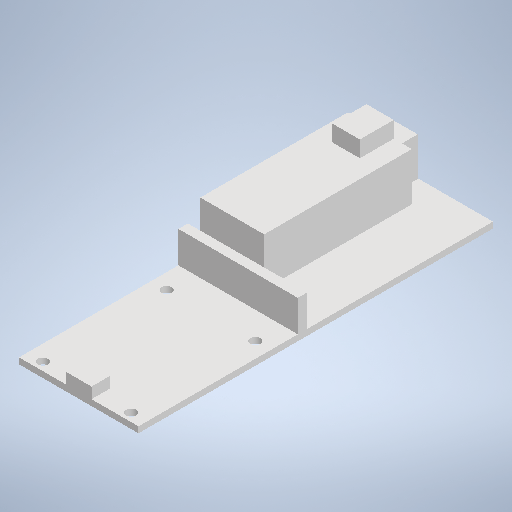
# Autodesk Inventor part: PCB Board
Saved by Autodesk Inventor 2025 (Build 290162000, 162)
## iProperties
Created: 2024-07-09
Part Number: PCB Board
Material: Generic
Document SubType Name: Modeling
Designer: track
Density: 1 g/cm^3
Appearance: Default
Author: track
Autodesk Inventor part; units mm, degrees
ref_plane "YZ Plane" through (0, 0, 0) normal (1, 0, 0) x (0, 1, 0)
ref_plane "XZ Plane" through (0, 0, 0) normal (0, 1, 0) x (-1, 0, 0)
ref_plane "XY Plane" through (0, 0, 0) normal (0, 0, 1) x (1, 0, 0)
sketch "Sketch1" plane through (0, 0, 0) normal (0, 1, 0) x (-1, 0, 0)
  line L0 (16.375, 48.6) -> (-16.375, 48.6)
  line L1 (-16.375, 48.6) -> (-16.375, -48.6)
  line L2 (-16.375, -48.6) -> (16.375, -48.6)
  line L3 (16.375, -48.6) -> (16.375, 48.6)
  line L4 (16.375, 48.6) -> (-16.375, -48.6) construction
  line L5 (-16.375, 48.6) -> (16.375, -48.6) construction
  point P0 (0, 0)
  dimension "d0" = 32.75
  dimension "d1" = 97.2
  constraints: 12 end point, 2 midpoint, 2 parallel, 1 horizontal, 1 perpendicular
  measures "d0" distance of L0.start L0.end
  measures "d1" distance of L0.end L1.end
extrude "Extrusion1" add sketch "Sketch1" along normal blind 1.65
sketch "Sketch3" plane through (0, 1.65, 0) normal (0, 1, 0) x (1, 0, 0)
  line L0 (-16.375, 48.6) -> (-16.375, -48.6) projected
  line L1 (-16.375, 41.6) -> (1.125, 41.6)
  line L2 (1.125, 41.6) -> (1.125, 1.1)
  line L3 (1.125, 1.1) -> (-16.375, 1.1)
  line L4 (-16.375, 1.1) -> (-16.375, 41.6)
  line L5 (16.375, 48.6) -> (-16.375, 48.6) projected
  point P0 (0, 0)
  dimension "d7" = 17.5
  dimension "d8" = 40.5
  dimension "d9" = 7
  constraints: 8 end point, 2 parallel, 1 horizontal, 1 perpendicular, 1 point on line
  measures "d7" distance of L1.start L1.end
  measures "d8" distance of L1.end L2.end
  measures "d9" distance between parallel lines of L5 L1
extrude "Extrusion3" add sketch "Sketch3" along normal blind 13.1
sketch "Sketch4" plane through (0, 1.65, 0) normal (0, 1, 0) x (1, 0, 0)
  line L0 (-16.375, 41.6) -> (1.125, 41.6) projected
  line L1 (-4.075, 41.6) -> (-11.075, 41.6)
  line L2 (-11.075, 41.6) -> (-11.075, 48.4118)
  line L3 (-11.075, 48.4118) -> (-4.075, 48.4118)
  line L4 (-4.075, 48.4118) -> (-4.075, 41.6)
  line L5 (-16.375, 48.6) -> (-16.375, 41.6) projected
  point P0 (0, 0)
  dimension "d12" = 7
  dimension "d13" = 5.3
  constraints: 8 end point, 2 parallel, 1 horizontal, 1 perpendicular, 1 point on line
  measures "d12" distance of L2.end L3.end
  measures "d13" distance between parallel lines of L5 L2
extrude "Extrusion4" add sketch "Sketch4" along normal blind 10.6
sketch "Sketch5" plane through (0, 14.75, 0) normal (0, 1, 0) x (1, 0, 0)
  line L0 (1.125, 41.6) -> (-16.375, 41.6) projected
  line L1 (-16.375, 41.6) -> (-16.375, 1.1) projected
  line L2 (-16.375, 1.1) -> (1.125, 1.1) projected
  line L3 (1.125, 1.1) -> (1.125, 41.6) projected
  line L4 (-11.075, 48.4118) -> (-11.075, 41.6) projected
  line L5 (-4.075, 41.6) -> (-11.075, 41.6) projected
  line L6 (-4.075, 41.6) -> (-4.075, 48.4118) projected
  line L7 (-4.075, 48.4118) -> (-11.075, 48.4118) projected
  line L8 (-4.075, 41.6) -> (-11.075, 41.6) projected
  line L9 (-3.825, 41.6) -> (-11.325, 41.6)
  line L10 (-11.325, 41.6) -> (-11.325, 32.3)
  line L11 (-11.325, 32.3) -> (-3.825, 32.3)
  line L12 (-3.825, 32.3) -> (-3.825, 41.6)
  point P0 (0, 0)
  point P1 (-7.575, 41.6)
  dimension "d16" = 9.3
  dimension "d17" = 7.5
  constraints: 8 end point, 2 midpoint, 2 parallel, 1 horizontal, 1 perpendicular, 1 point on line
  measures "d16" distance of L11.end L9.start
  measures "d17" distance of L10.end L11.end
extrude "Extrusion5" add sketch "Sketch5" along normal blind 4.46 contours L12 L11 L10 L0
sketch "Sketch6" plane through (-4.075, 1.65, -48.4118) normal (0, 0, -1) x (-1, 0, 0)
  point P0 (-4.075, -1.65)
sketch "Sketch7" plane through (0, 1.65, 0) normal (0, 1, 0) x (1, 0, 0)
  line L0 (-11.325, 32.3) -> (-11.325, 41.6) projected
  line L1 (-11.325, 41.6) -> (-16.375, 41.6) projected
  line L2 (-16.375, 41.6) -> (-16.375, 1.1) projected
  line L3 (-16.375, 1.1) -> (1.125, 1.1) projected
  line L4 (1.125, 1.1) -> (1.125, 41.6) projected
  line L5 (1.125, 41.6) -> (-3.825, 41.6) projected
  line L6 (-3.825, 41.6) -> (-3.825, 32.3) projected
  line L7 (-3.825, 32.3) -> (-11.325, 32.3) projected
  line L8 (16.375, -48.6) -> (16.375, 48.6) projected
  line L9 (-16.375, 48.6) -> (-16.375, -48.6) projected
  line L10 (16.375, -2.3) -> (-16.375, -2.3)
  line L11 (-16.375, -2.3) -> (-16.375, -4.9)
  line L12 (-16.375, -4.9) -> (16.375, -4.9)
  line L13 (16.375, -4.9) -> (16.375, -2.3)
  point P0 (0, 0)
  point P1 (-16.375, -2.3)
  dimension "d20" = 2.6
  dimension "d21" = 3.4
  constraints: 8 end point, 2 parallel, 2 point on line, 1 horizontal, 1 perpendicular
  measures "d20" distance between parallel lines of L10 L12
  measures "d21" distance between parallel lines of L3 L10
extrude "Extrusion6" add sketch "Sketch7" along normal blind 8.65 contours L10 L8 L12 L9
sketch "Sketch8" plane through (0, 1.65, 0) normal (0, 1, 0) x (1, 0, 0)
  circle A0 centre (-12.125, -46.35) radius 1.4
  line L0 (-16.375, -4.9) -> (-16.375, -48.6) projected
  line L1 (-16.375, -48.6) -> (16.375, -48.6) projected
  circle A1 centre (-12.125, -12.35) radius 1.4
  line L2 (0, -48.6) -> (0, 0) construction
  circle A2 centre (12.125, -46.35) radius 1.4
  circle A3 centre (12.125, -12.35) radius 1.4
  dimension "d24" = 2.8
  dimension "d25" = 4.25
  dimension "d26" = 2.25
  dimension "d27" = 34
  constraints: 4 centre point, 2 end point, 2 symmetric about line, 1 equal radius, 1 midpoint, 1 vertical, 2 other
  measures "d24" diameter of A0
  measures "d25" distance from line of L0 A0.centre
  measures "d26" distance from line of L1 A0.centre
  measures "d27" distance of A1.centre A0.centre
extrude "Extrusion7" cut sketch "Sketch8" against normal up to surface (1.65 mm away)
sketch "Sketch9" plane through (0, 1.65, 0) normal (0, 1, 0) x (1, 0, 0)
  line L0 (-16.375, -48.6) -> (16.375, -48.6) projected
  line L1 (3.5, -43.6) -> (-3.5, -43.6)
  line L2 (-3.5, -43.6) -> (-3.5, -48.6)
  line L3 (-3.5, -48.6) -> (3.5, -48.6)
  line L4 (3.5, -48.6) -> (3.5, -43.6)
  line L5 (3.5, -43.6) -> (-3.5, -48.6) construction
  line L6 (-3.5, -43.6) -> (3.5, -48.6) construction
  point P0 (0, 0)
  point P1 (0, -46.1)
  point P2 (0, -48.6)
  dimension "d30" = 5
  dimension "d31" = 7
  constraints: 12 end point, 4 midpoint, 2 parallel, 1 horizontal, 1 perpendicular, 1 point on line
  measures "d30" distance of L1.end L2.end
  measures "d31" distance of L1.start L1.end
extrude "Extrusion8" add sketch "Sketch9" along normal blind 3
body "Solid1"
